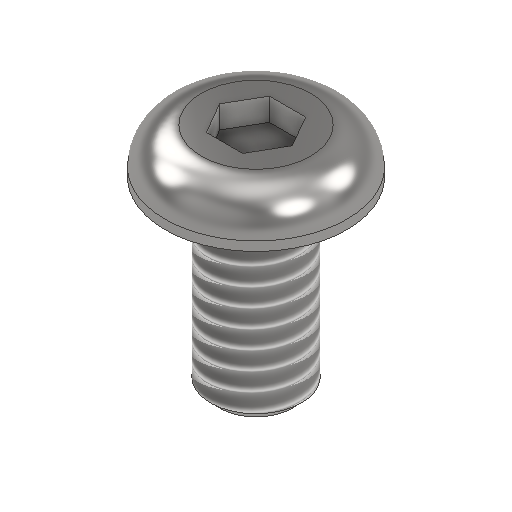
# Autodesk Inventor part: M2-4_screw
Saved by Autodesk Inventor 2026.2 (Build 302298000, 298)
## iProperties
Created: 2026-03-19
Part Number: M2-4_screw
Material: ステンレス鋼 440C
Document SubType Name: Modeling
Designer: zetsu
Density: 7.75 g/cm^3
Appearance: 半つや出し
Author: zetsu
Autodesk Inventor part; units mm, degrees
ref_plane "YZ Plane" through (0, 0, 0) normal (1, 0, 0) x (0, 1, 0)
ref_plane "XZ Plane" through (0, 0, 0) normal (0, 1, 0) x (-1, 0, 0)
ref_plane "XY Plane" through (0, 0, 0) normal (0, 0, 1) x (1, 0, 0)
sketch "スケッチ1" plane through (0, 0, 0) normal (0, 1, 0) x (-1, 0, 0)
  circle A0 centre (0, 0) radius 2
  dimension "d0" = 4
  constraints: 1 centre point, 1 coincident
  measures "d0" diameter of A0
extrude "押し出し1" add sketch "スケッチ1" against normal blind 1
sketch "スケッチ2" plane through (0, -1, 0) normal (0, -1, 0) x (1, 0, 0)
  circle A0 centre (0, 0) radius 1
  dimension "d3" = 2
  constraints: 1 centre point, 1 coincident
  measures "d3" diameter of A0
extrude "押し出し2" add sketch "スケッチ2" along normal blind 4
chamfer "面取り1" distance 0.2 angle 45 1 edges at (-1, -5, 0)
fillet "フィレット1" radius 0.8 1 edges at (2, 0, 0)
thread "ねじ1" size "M2x0.4" class "6g" standard "ANSI Metric M Profile" full length
sketch "スケッチ3" plane through (0, 0, 0) normal (0, 1, 0) x (1, 0, 0)
  circle A0 centre (0, 0) radius 0.8 projected
  line L0 (-0.8, 0) -> (-0.4, 0.6928)
  line L1 (-0.8, 0) -> (0, 0) construction
  line L2 (-0.4, -0.6928) -> (-0.8, 0)
  line L3 (0.4, -0.6928) -> (-0.4, -0.6928)
  line L4 (0.8, 0) -> (0.4, -0.6928)
  line L5 (0.4, 0.6928) -> (0.8, 0)
  line L6 (-0.4, 0.6928) -> (0.4, 0.6928)
  point P0 (0.8, 0)
  dimension "d12" = 0.8
  dimension "d13" = 60
  dimension "d16" = 360
  constraints: 14 end point, 1 equal length, 1 horizontal, 1 horizontal alignment, 20 other
  measures "d12" distance of L0.start L0.end
  measures "d13" angle of L1 L0
extrude "押し出し3" cut sketch "スケッチ3" against normal blind 0.5 contours L4 L3 L2 L0 L6 L5
